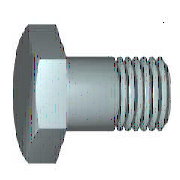
# Autodesk Inventor part: CNS 4321 - M12 x 150
Saved by Autodesk Inventor 2017 SP1 (Build 210196100, 196)
## iProperties
IsCustomPart: 0
Created: 2016-02-22
Part Number: CNS 4321 - M12 x 150
Material: Steel, Mild
Description: Hex-Head Bolt
Document SubType Name: Modeling
Standard: CNS 4321
Designer: Zach
Standards Organization: CNS
Language: en-US
Size Designation: M12 x 150
Categories: <MemberInstance><Categories><Category DisplayName="Fasteners" InternalName="e4da775c-781d-43d5-af7c-5136215cf5a6" Mnemonic="FSTN"><Category DisplayName="Bolts" InternalName="536e6df0-f778-49ac-b2f2-25c71d2aa0b2" Mnemonic="SCRW"><CategoryParameter DisplayName="Nominal Diameter Designation" InternalName="03caf894-eafd-4c09-a035-916ac084b87b" Mnemonic="nomdiadesig"/><CategoryParameter DisplayName="Nominal Length" InternalName="238ecbaf-3e6c-45dd-aa95-4068c8e0fd02" Mnemonic="nomlen"/><CategoryParameter DisplayName="Thread Designation" InternalName="586d5e89-370a-4089-914f-0110033585c7" Mnemonic="thrdesign"/><CategoryParameter DisplayName="Thread Series Designation" InternalName="87c5849c-b3a5-4c3e-9c9b-2feecef9be86" Mnemonic="thrserdsgn"/><CategoryParameter DisplayName="Nominal Diameter" InternalName="8bbe3f8e-44cf-40a9-a251-3a6edc8168d6" Mnemonic="nomdia"/><CategoryParameter DisplayName="Thread Type" InternalName="b4bbb7bc-d6aa-4c9f-a9a9-4152b9f6fe49" Mnemonic="thrtype"/><CategoryParameter DisplayName="Thread Pitch" InternalName="bb82302e-82d8-4176-8fc1-c5d7bb17d5ad" Mnemonic="pitch1"/><CategoryParameter DisplayName="Threads per Unit" InternalName="bdc6e7d2-ffd0-4d9c-a173-16b95ebb912d" Mnemonic="thrperunit1"/><CategoryParameter DisplayName="Thread Class" InternalName="ebc0d23b-2cc6-4d2a-b376-d52aae53bab6" Mnemonic="thrclss"/><Category DisplayName="Hex Head" InternalName="520da9a1-ead7-4898-b571-59b4b339a5c6" Mnemonic="PLSCRW"><CategoryParameter DisplayName="Grip Length" InternalName="14b808f1-b175-4f80-b2c8-3c2ac1acde4c" Mnemonic="grplen"/><CategoryParameter DisplayName="Width Across Flats" InternalName="1cb53529-b7fd-49c5-a5c5-85a22d509c9e" Mnemonic="waflat"/><CategoryParameter DisplayName="Head Height" InternalName="3a45ce7b-b38d-4f77-aad7-a2328eea5aef" Mnemonic="headh"/><CategoryParameter DisplayName="Thread Length" InternalName="50b9771a-9fb7-48bc-803b-80099da79f2d" Mnemonic="thrlen"/><CategoryParameter DisplayName="Width Across Corners" InternalName="a21dc55e-7dbc-4faf-83dd-c7c1bfd07428" Mnemonic="wacor"/><CategoryParameter DisplayName="Shank Diameter" InternalName="bad16e07-a90c-44cc-a6af-8a6b56171876" Mnemonic="grpdia"/><CategoryParameter DisplayName="Diameter of Contact Area" InternalName="cc3b219b-8087-4820-96e9-69a08f47c1a6" Mnemonic="conardia"/></Category></Category></Category><Category DisplayName="DataType" InternalName="23b78d0f-2648-40c6-8793-ca6db495c9e8" Mnemonic="DATATYPE"><CategoryParameter DisplayName="DisplayName" InternalName="05415f3d-3907-474b-a020-eb9d644f4cf3" Mnemonic="DISPLAYNAME"/><CategoryParameter DisplayName="Standard" InternalName="0c0a119c-1e12-4c84-803f-101930972f5e" Mnemonic="STANDARD"/><CategoryParameter DisplayName="Description" InternalName="13903e3d-64b1-4950-80da-f627842ea37f" Mnemonic="DESCRIPTION"/><CategoryParameter DisplayName="Designation" InternalName="2675968c-4ce5-49e0-a4f5-552d29089031" Mnemonic="DESIGNATION"/><CategoryParameter DisplayName="Default Row" InternalName="2af9ec52-faaa-4026-b378-f9fa4afca842" Mnemonic="DEFAULTROW"/><CategoryParameter DisplayName="Folder Name" InternalName="3f06958e-8713-4116-9be7-ed6184ecc97b" Mnemonic="FOLDERNAME"/><CategoryParameter DisplayName="Revision Guid" InternalName="45a75005-10b1-4dfc-8d6d-dfe629f0b93c" Mnemonic="REVISIONGUID"/><CategoryParameter DisplayName="FileName" InternalName="8b46a4cc-9585-4fed-90c3-899f57e09a73" Mnemonic="FILENAME"/><CategoryParameter DisplayName="StdsOrg" InternalName="8f5914e1-4693-403f-8ab5-d37768198c9d" Mnemonic="STDSORG"/><CategoryParameter DisplayName="Family Version" InternalName="914462f6-6e19-4b14-ba84-155b9680b1d0" Mnemonic="FAMILYREVISION"/><CategoryParameter DisplayName="Standard Revision" InternalName="91d5a463-65c2-4fde-b823-3b7fea5e8e17" Mnemonic="STANDARDREVISION"/><CategoryParameter DisplayName="Member Revision" InternalName="a65d44b9-392f-4f4f-857b-e4b3d54996fe" Mnemonic="MEMBERREVISION"/><CategoryParameter DisplayName="ClipFormat" InternalName="bc51e27b-3422-4e78-93ef-cec197ddf230" Mnemonic="CLIPFORMAT"/><CategoryParameter DisplayName="Manufacturer" InternalName="cd6c7a72-a28a-4e50-99a9-2c7f4e13e5ad" Mnemonic="MANUFACTURER"/><CategoryParameter DisplayName="InternalName" InternalName="cf1d0246-76d9-4b4a-8305-fa0409afb5c1" Mnemonic="INTERNALNAME"/><CategoryParameter DisplayName="IsMetric" InternalName="e2385c5b-1ea4-4823-96a8-8de651266ec3" Mnemonic="ISMETRIC"/><Category DisplayName="Part" InternalName="c0e0b642-3bcb-4cc8-9e80-f96d35c4afa4" Mnemonic="PART"><CategoryParameter DisplayName="Part Number" InternalName="016b6077-bfbe-49bd-92c9-d8d59c39c941" Mnemonic="PARTNUMBER"/><CategoryParameter DisplayName="Stock Number" InternalName="4dba7c1c-e26c-444e-836c-b08b433409a8" Mnemonic="STOCKNUMBER"/><CategoryParameter DisplayName="Material Key" InternalName="5c9a8adb-dd2b-4535-b97f-0a94a95fe41f" Mnemonic="MATERIALKEY"/><CategoryParameter DisplayName="Material" InternalName="818a152a-d3c3-49ca-80ee-df7d91421b8e" Mnemonic="MATERIAL"/></Category></Category><Category DisplayName="LegacyMap" InternalName="cd87c42b-3e48-431e-b5c0-1cbeb14dfe77" Mnemonic="LEGACYMAP"><CategoryParameter DisplayName="unique DA member ID" InternalName="0918ad47-427f-4fed-ae26-24c81c58f590" Mnemonic="DACOOKIE"/><CategoryParameter DisplayName="Merge11 ID" InternalName="0ee8fb18-e2ed-4f39-96f6-1f4b5f50aa71" Mnemonic="MERGE11"/><CategoryParameter DisplayName="unique CC member ID" InternalName="5193edd4-b2b0-4ab4-9d54-de900eee34e0" Mnemonic="CCCOOKIE"/><CategoryParameter DisplayName="Split ID" InternalName="72b5c83c-be7f-45c4-ae51-9160ea6deb26" Mnemonic="SPLIT"/><CategoryParameter DisplayName="MemberID" InternalName="8e5e0294-fc51-4c8f-b3d7-003dc5ed94f6" Mnemonic="MEMBERID"/><CategoryParameter DisplayName="CatalogName" InternalName="d99d1e27-aa94-4de2-af4c-c348882a6f4f" Mnemonic="CATALOGNAME"/><CategoryParameter DisplayName="FamilyNumber" InternalName="e705e1f4-09cb-413e-91f9-551b4188271e" Mnemonic="FAMILYNUMBER"/></Category></Categories><FamilyTemplate Id="si0002"><FamilyTemplateParameters><FamilyTemplateParameter ObjectType="kUserParameterObject" ValueType="xs:double" Id="1" ObjectReferenceKey="GUL"/><FamilyTemplateParameter ObjectType="kUserParameterObject" ValueType="xs:double" Id="2" ObjectReferenceKey="SPD"/><FamilyTemplateParameter ObjectType="kUserParameterObject" ValueType="xs:double" Id="3" ObjectReferenceKey="NLG"/><FamilyTemplateParameter ObjectType="kUserParameterObject" ValueType="xs:double" Id="4" ObjectReferenceKey="GD"/><FamilyTemplateParameter ObjectType="kUserParameterObject" ValueType="xs:double" Id="5" ObjectReferenceKey="TPU"/><FamilyTemplateParameter ObjectType="kUserParameterObject" ValueType="xs:double" Id="6" ObjectReferenceKey="WFT"/><FamilyTemplateParameter ObjectType="kUserParameterObject" ValueType="xs:double" Id="7" ObjectReferenceKey="GD1"/><FamilyTemplateParameter ObjectType="kUserParameterObject" ValueType="xs:double" Id="8" ObjectReferenceKey="GEL"/><FamilyTemplateParameter ObjectType="kUserParameterObject" ValueType="xs:double" Id="9" ObjectReferenceKey="SW"/><FamilyTemplateParameter ObjectType="kUserParameterObject" ValueType="xs:double" Id="10" ObjectReferenceKey="THREADDIA"/><FamilyTemplateParameter ObjectType="kUserParameterObject" ValueType="xs:double" Id="11" ObjectReferenceKey="SDH"/><FamilyTemplateParameter ObjectType="kUserParameterObject" ValueType="xs:double" Id="12" ObjectReferenceKey="ANG1"/><FamilyTemplateParameter ObjectType="kUserParameterObject" ValueType="xs:double" Id="13" ObjectReferenceKey="TOA"/><FamilyTemplateParameter ObjectType="kUserParameterObject" ValueType="xs:double" Id="14" ObjectReferenceKey="BDM"/><FamilyTemplateParameter ObjectType="kUserParameterObject" ValueType="xs:double" Id="15" ObjectReferenceKey="RR"/><FamilyTemplateParameter ObjectType="kUserParameterObject" ValueType="xs:double" Id="16" ObjectReferenceKey="KOH"/><FamilyTemplateParameter ObjectType="kUserParameterObject" ValueType="xs:double" Id="17" ObjectReferenceKey="PTC"/><FamilyTemplateParameter ObjectType="kUserParameterObject" ValueType="xs:double" Id="18" ObjectReferenceKey="NND"/><FamilyTemplateParameter ObjectType="kUserParameterObject" ValueType="xs:double" Id="19" ObjectReferenceKey="SW0"/><FamilyTemplateParameter ObjectType="kUserParameterObject" ValueType="xs:double" Id="20" ObjectReferenceKey="GAL"/><FamilyTemplateParameter ObjectType="kUserParameterObject" ValueType="xs:double" Id="21" ObjectReferenceKey="SD"/><FamilyTemplateParameter ObjectType="kUserParameterObject" ValueType="xs:double" Id="22" ObjectReferenceKey="SD2"/><FamilyTemplateParameter ObjectType="kUserParameterObject" ValueType="xs:double" Id="23" ObjectReferenceKey="E0"/><FamilyTemplateParameter ObjectType="kPropertyObject" ValueType="xs:string" Id="100" ObjectReferenceKey="{32853F0F-3444-11d1-9E93-0060B03C1CA6}" SubObjectId="52"/><FamilyTemplateParameter ObjectType="kPropertyObject" ValueType="xs:string" Id="105" ObjectReferenceKey="{32853F0F-3444-11d1-9E93-0060B03C1CA6}" SubObjectId="5"/><FamilyTemplateParameter ObjectType="kPartComponentDefinitionObject" ValueType="xs:string" Id="110" SubObjectId="Material"/><FamilyTemplateParameter ObjectType="kThreadFeatureObject" ValueType="xs:structure" Id="300" ObjectReferenceKey="100200001000000049150000000000008000000000000000" SubObjectId="ThreadInfo"><FamilyTemplateParameter ObjectType="" ValueType="xs:string" Id="301" SubObjectId="ThreadDesignation"/><FamilyTemplateParameter ObjectType="" ValueType="xs:string" Id="302" SubObjectId="ThreadType"/><FamilyTemplateParameter ObjectType="" ValueType="xs:string" Id="303" SubObjectId="ThreadClass"/></FamilyTemplateParameter></FamilyTemplateParameters></FamilyTemplate><CategoryParameterMap><ParamToTemplateMap><ParamToTemplate CategoryParameter="//CategoryParameter[@InternalName='05415f3d-3907-474b-a020-eb9d644f4cf3']" ConstantValue="CNS 4321"/><ParamToTemplate CategoryParameter="//CategoryParameter[@InternalName='cf1d0246-76d9-4b4a-8305-fa0409afb5c1']" ConstantValue="cf93c8bf-f13b-41ae-b581-fd96f20db1c8"/><ParamToTemplate CategoryParameter="//CategoryParameter[@InternalName='3f06958e-8713-4116-9be7-ed6184ecc97b']" ConstantValue="CNS 4321"/><ParamToTemplate CategoryParameter="//CategoryParameter[@InternalName='914462f6-6e19-4b14-ba84-155b9680b1d0']" ConstantValue="10"/><ParamToTemplate CategoryParameter="//CategoryParameter[@InternalName='bc51e27b-3422-4e78-93ef-cec197ddf230']" ConstantValue="CF_INVENTOR.STDPARTS"/><ParamToTemplate CategoryParameter="//CategoryParameter[@InternalName='e2385c5b-1ea4-4823-96a8-8de651266ec3']" ConstantValue="true"/><ParamToTemplate CategoryParameter="//CategoryParameter[@InternalName='13903e3d-64b1-4950-80da-f627842ea37f']" ConstantValue="Hex-Head Bolt"/><ParamToTemplate CategoryParameter="//CategoryParameter[@InternalName='8f5914e1-4693-403f-8ab5-d37768198c9d']" ConstantValue="CNS"/><ParamToTemplate CategoryParameter="//CategoryParameter[@InternalName='0c0a119c-1e12-4c84-803f-101930972f5e']" ConstantValue="CNS 4321"/><ParamToTemplate CategoryParameter="//CategoryParameter[@InternalName='cd6c7a72-a28a-4e50-99a9-2c7f4e13e5ad']" TemplateParameter="104"/><ParamToTemplate CategoryParameter="//CategoryParameter[@InternalName='91d5a463-65c2-4fde-b823-3b7fea5e8e17']" TemplateParameter="103"/><ParamToTemplate CategoryParameter="//CategoryParameter[@InternalName='45a75005-10b1-4dfc-8d6d-dfe629f0b93c']" ConstantValue="aa53406d-8931-4ce5-8203-952556d26351"/><ParamToTemplate CategoryParameter="//CategoryParameter[@InternalName='2af9ec52-faaa-4026-b378-f9fa4afca842']" ConstantValue="10"/><ParamToTemplate CategoryParameter="//CategoryParameter[@InternalName='d99d1e27-aa94-4de2-af4c-c348882a6f4f']" ConstantValue="CNS"/><ParamToTemplate CategoryParameter="//CategoryParameter[@InternalName='e705e1f4-09cb-413e-91f9-551b4188271e']" ConstantValue="13"/><ParamToTemplate CategoryParameter="//CategoryParameter[@InternalName='8b46a4cc-9585-4fed-90c3-899f57e09a73']" ConstantValue="CNS 4321 - M12 x 1.25 x 150"/><ParamToTemplate CategoryParameter="//CategoryParameter[@InternalName='a65d44b9-392f-4f4f-857b-e4b3d54996fe']" ConstantValue="44f10b6c-01e0-42d0-baf4-a774f2d83866"/><ParamToTemplate CategoryParameter="//CategoryParameter[@InternalName='14b808f1-b175-4f80-b2c8-3c2ac1acde4c']" ConstantValue="4"/><ParamToTemplate CategoryParameter="//CategoryParameter[@InternalName='ebc0d23b-2cc6-4d2a-b376-d52aae53bab6']" ConstantValue="6g"/><ParamToTemplate CategoryParameter="//CategoryParameter[@InternalName='b4bbb7bc-d6aa-4c9f-a9a9-4152b9f6fe49']" ConstantValue="ISO Metric profile"/><ParamToTemplate CategoryParameter="//CategoryParameter[@InternalName='8e5e0294-fc51-4c8f-b3d7-003dc5ed94f6']" ConstantValue="1200"/><ParamToTemplate CategoryParameter="//CategoryParameter[@InternalName='bad16e07-a90c-44cc-a6af-8a6b56171876']" TemplateParameter="14"/><ParamToTemplate CategoryParameter="//CategoryParameter[@InternalName='2675968c-4ce5-49e0-a4f5-552d29089031']" TemplateParameter="100"/><ParamToTemplate CategoryParameter="//CategoryParameter[@InternalName='a21dc55e-7dbc-4faf-83dd-c7c1bfd07428']" TemplateParameter="23"/><ParamToTemplate CategoryParameter="//CategoryParameter[@InternalName='50b9771a-9fb7-48bc-803b-80099da79f2d']" TemplateParameter="8"/><ParamToTemplate CategoryParameter="//CategoryParameter[@InternalName='3a45ce7b-b38d-4f77-aad7-a2328eea5aef']" TemplateParameter="16"/><ParamToTemplate CategoryParameter="//CategoryParameter[@InternalName='818a152a-d3c3-49ca-80ee-df7d91421b8e']" TemplateParameter="110"/><ParamToTemplate CategoryParameter="//CategoryParameter[@InternalName='238ecbaf-3e6c-45dd-aa95-4068c8e0fd02']" TemplateParameter="3"/><ParamToTemplate CategoryParameter="//CategoryParameter[@InternalName='8bbe3f8e-44cf-40a9-a251-3a6edc8168d6']" TemplateParameter="18"/><ParamToTemplate CategoryParameter="//CategoryParameter[@InternalName='016b6077-bfbe-49bd-92c9-d8d59c39c941']" TemplateParameter="105"/><ParamToTemplate CategoryParameter="//CategoryParameter[@InternalName='bb82302e-82d8-4176-8fc1-c5d7bb17d5ad']" TemplateParameter="17"/><ParamToTemplate CategoryParameter="//CategoryParameter[@InternalName='586d5e89-370a-4089-914f-0110033585c7']" TemplateParameter="301"/><ParamToTemplate CategoryParameter="//CategoryParameter[@InternalName='bdc6e7d2-ffd0-4d9c-a173-16b95ebb912d']" TemplateParameter="5"/></ParamToTemplateMap></CategoryParameterMap></MemberInstance>
Density: 7.85 g/cm^3
Appearance: Semi-Polished
Author: Zach
Autodesk Inventor part; units mm, degrees
ref_plane "YZ Plane" through (0, 0, 0) normal (1, 0, 0) x (0, 1, 0)
ref_plane "XZ Plane" through (0, 0, 0) normal (0, 1, 0) x (-1, 0, 0)
sketch "Sketch1" plane through (0, 0, 0) normal (0, 0, 1) x (1, 0, 0)
  line L0 (0, 9.5) -> (0, 6)
  line L1 (4, 6) -> (150, 6)
  line L2 (150, 6) -> (150, 0)
  line L3 (150, 0) -> (-0.4001, 0)
  line L4 (-30.4801, 0) -> (180.08, 0) projected
  line L5 (-0.4001, 0) -> (-0.4001, 9.5)
  line L6 (-0.4001, 9.5) -> (0, 9.5)
  line L7 (4, 6) -> (3.2331, 6)
  line L8 (3.2331, 6) -> (0, 6)
  line L9 (0, -1.9) -> (0, 11.4) projected
  dimension "d0" = 150
  dimension "d1" = 146
  dimension "d2" = 12
  dimension "d9" = 0.4001
  dimension "d10" = 19
  dimension "d13" = 0.7669
  dimension "d14" = 12
  constraints: 16 end point, 2 collinear, 2 perpendicular, 1 parallel
  measures "d0" distance between parallel lines of L2 L0
  measures "d1" distance from line of L1.start L2
  measures "d2" diameter of L1 L3
  measures "d9" distance between parallel lines of L5 L0
  measures "d10" diameter of L6 L3
  measures "d13" distance of L1.start L7.end
  measures "d14" diameter of L8 L3
revolve "Body" add sketch "Sketch1" angle 360 about axis through (150, 0, 0) along (-1, 0, 0)
sketch "Sketch2" plane through (-0.4001, 0, 0) normal (-1, 0, 0) x (0, 0, 1)
  line L0 (0, 10.9697) -> (9.5, 5.4848)
  line L1 (9.5, 5.4848) -> (9.5, -5.4848)
  line L2 (9.5, -5.4848) -> (0, -10.9697)
  line L3 (0, -10.9697) -> (-9.5, -5.4848)
  line L4 (-9.5, -5.4848) -> (-9.5, 5.4848)
  line L5 (-9.5, 5.4848) -> (0, 10.9697)
  point P0 (0, 0)
  point P1 (0, 0)
  dimension "d11" = 19
  constraints: 12 end point, 1 coincident, 1 vertical, 11 other
  measures "d11" distance between parallel lines of L4 L1
extrude "Head" add sketch "Sketch2" along normal blind 7.6
sketch "Sketch4" plane through (0, 0, 0) normal (0, 0, 1) x (1, 0, 0)
  line L0 (-8.0001, 9.5) -> (-8.0001, 10.9697)
  line L1 (-8.0001, 10.9697) -> (-7.1516, 10.9697)
  line L2 (-7.1516, 10.9697) -> (-8.0001, 9.5)
  line L3 (-9.5201, 0) -> (1.1199, 0) projected
  line L4 (-0.4001, 10.9697) -> (-8.0001, 10.9697) projected
  line L5 (-8.0001, 5.4848) -> (-8.0001, 10.9697) projected
  dimension "d5" = 30
  dimension "d19" = 19
  constraints: 6 end point, 2 collinear, 1 perpendicular, 1 vertical
  measures "d5" angle of L2 L0
  measures "d19" diameter of L0.start L3
revolve "Chamfer1" cut sketch "Sketch4" angle 360 about axis through (-10, 0, 0) along (1, 0, 0)
thread "Thread" size "M12x1.25" class "6g" standard "ISO Metric profile" length 146
chamfer "Chamfer2" distance 0.7668 distance2 0.7669 1 edges at (150, -6, 0) measured on face at (150, -1.326, -0.0818)
ref_plane "Work Plane1" through (1.525, 0, 0) normal (0, 0, 1) x (1, 0, 0)
equation "\"d0\" = NLG"
equation "\"d1\" = GEL"
equation "\"d2\" = GD"
equation "\"d10\" = SD2"
equation "\"d14\" = BDM"
equation "\"d11\" = SW"
equation "\"d3\" = KOH - SD"
equation "\"d5\" = ANG1"
equation "\"d19\" = SW0"
equation "\"d15\" = GEL"
equation "\"d6\" = -0.5 * SPD + 0.5 * GD"
equation "\"NLG\" = 150"
equation "\"GD\" = NND"
equation "\"BDM\" = NND"
equation "\"KOH\" = 8"
equation "\"GEL\" = 146"
equation "\"SW\" = 19"
equation "\"SW0\" = SW"
equation "\"SPD\" = NND - 1.2269 * PTC"
equation "\"SD2\" = SW"
equation "\"SD\" = WFT"
equation "\"ANG1\" = 30deg"
equation "\"GAL\" = 0.61345 * PTC"
equation "\"GUL\" = 0.61345 * PTC"
equation "\"RR\" = 0.6"
equation "\"WFT\" = 0.4"
equation "\"GD1\" = THREADDIA - 1.2269 * PTC"
equation "\"THREADDIA\" = 12"
equation "\"SDH\" = SW"
equation "\"TOA\" = 30deg"
equation "\"PTC\" = 1.25"
equation "\"NND\" = 12"
equation "\"E0\" = 1.155 * SW"
body "Solid1"
